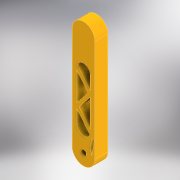
# Autodesk Inventor part: EslabonRodillaCadera
Saved by Autodesk Inventor 2021 (Build 250183000, 183)
## iProperties
Created: 2024-02-25
Part Number: EslabonRodillaCadera
Material: PLA
Document SubType Name: Modeling
Designer: Martin
Density: 1.27 g/cm^3
Appearance: PLA
Mass: 95.6941 g
Surface Area: 224.769 cm^2
Volume: 75.3497 cm^3
Author: Martin
Autodesk Inventor part; units mm, degrees
ref_plane "YZ Plane" through (0, 0, 0) normal (1, 0, 0) x (0, 1, 0)
ref_plane "XZ Plane" through (0, 0, 0) normal (0, 1, 0) x (-1, 0, 0)
ref_plane "XY Plane" through (0, 0, 0) normal (0, 0, 1) x (1, 0, 0)
sketch "Sketch1" plane through (0, 0, 0) normal (0, 0, 1) x (1, 0, 0)
  line L0 (0.0065, 157) -> (0.0065, 0) construction
  line L1 (-17.4935, 157) -> (-17.4935, 0)
  line L2 (17.5065, 0) -> (17.5065, 157)
  arc A0 (17.5065, 157) -> (-17.4935, 157) centre (0.0065, 157) ccw
  arc A1 (-17.4935, 0) -> (17.5065, 0) centre (0.0065, 0) ccw
  circle A2 centre (0.0065, 0) radius 11.1
  circle A3 centre (0.0065, 157) radius 7.5
  line L3 (4.0065, 157) -> (4.0065, 135)
  line L4 (4.0065, 135) -> (-3.9935, 135)
  line L5 (-3.9935, 135) -> (-3.9935, 157)
  line L6 (-3.9935, 157) -> (4.0065, 157)
  line L7 (0.0065, 157.5) -> (0.0065, -30.5)
  line L8 (0.0065, 157) -> (5.7519, 152.1791)
  line L9 (0.0065, 157) -> (0.0065, 149.5) construction
  arc A4 (5.7519, 152.1791) -> (4.0065, 147.4936) centre (13.9526, 146.4565) ccw
  line L10 (0.0065, 157) -> (-5.7388, 152.1791)
  arc A5 (-3.9935, 147.4936) -> (-5.7388, 152.1791) centre (-13.9395, 146.4565) ccw
  line L11 (0.0065, 157.5) -> (0.0065, 133.5) construction
  line L12 (4.0065, 157.5) -> (4.0065, 133.5)
  line L13 (-3.9935, 133.5) -> (-3.9935, 157.5)
  arc A6 (4.0065, 157.5) -> (-3.9935, 157.5) centre (0.0065, 157.5) ccw
  arc A7 (-3.9935, 133.5) -> (4.0065, 133.5) centre (0.0065, 133.5) ccw
  point P0 (0.0065, 157)
  point P1 (-3.9935, 147.4936)
  point P2 (0.0065, 145.5)
  dimension "d38" = 15
  dimension "d19" = 35
  dimension "d20" = 22.2
  dimension "d39" = 22
  dimension "d40" = 8
  dimension "d41" = 4
  dimension "d42" = 4
  dimension "d43" = 50
  dimension "d44" = 5
  dimension "d45" = 10
  dimension "d50" = 24
  dimension "d59" = 157
  constraints: 32 end point, 12 point on circle, 8 tangent, 7 centre point, 4 parallel, 2 point on line, 1 coincident, 1 equal length, 1 midpoint, 1 perpendicular, 1 vertical, 3 other
  measures "d19" diameter of A1
  measures "d20" diameter of A2
  measures "d39" distance of L5.start L5.end
  measures "d40" distance of L3.end L5.start
  measures "d41" distance between parallel lines of L5 L7
  measures "d42" distance between parallel lines of L7 L3
  measures "d43" angle of L9 L8
  measures "d44" distance of L8.end A4.end
  measures "d45" radius of A4
  measures "d50" distance of L7.start L11.end
  measures "d59" distance of L0.end L0.start
extrude "Extrusion1" add sketch "Sketch1" along normal mid plane 6
sketch "Sketch6" plane through (0, 0, 3) normal (0, 0, 1) x (1, 0, 0)
  arc A0 (-17.4935, 0) -> (17.5065, 0) centre (0.0065, 0) ccw projected
  line L0 (17.5065, 0) -> (17.5065, 157) projected
  arc A1 (17.5065, 157) -> (-17.4935, 157) centre (0.0065, 157) ccw projected
  line L1 (-17.4935, 157) -> (-17.4935, 0) projected
  arc A2 (-3.9935, 133.5) -> (4.0065, 133.5) centre (0.0065, 133.5) ccw projected
  line L2 (-3.9935, 133.5) -> (-3.9935, 147.4936) projected
  arc A3 (-3.9935, 147.4936) -> (-5.7388, 152.1791) centre (-13.9395, 146.4565) ccw projected
  arc A4 (5.7519, 152.1791) -> (-5.7388, 152.1791) centre (0.0065, 157) ccw projected
  arc A5 (5.7519, 152.1791) -> (4.0065, 147.4936) centre (13.9526, 146.4565) ccw projected
  line L3 (4.0065, 147.4936) -> (4.0065, 133.5) projected
  circle A6 centre (0.0065, 0) radius 11.1 projected
  point P0 (0, 0)
extrude "Extrusion4" add sketch "Sketch6" along normal blind 2 contours L1 A1 L0 A0 | L2 A3 A4 A5 L3 A2
sketch "Sketch7" plane through (0, 0, 5) normal (0, 0, 1) x (1, 0, 0)
  line L0 (0, 244.3) -> (0, -244.3) projected
  line L1 (17.5065, 0) -> (17.5065, 157) projected
  arc A0 (17.5065, 157) -> (-17.4935, 157) centre (0.0065, 157) ccw projected
  line L2 (-17.4935, 157) -> (-17.4935, 0) projected
  arc A1 (-17.4935, 0) -> (17.5065, 0) centre (0.0065, 0) ccw projected
  circle A2 centre (0.0065, 0) radius 11.1 projected
  circle A3 centre (0.0065, 0) radius 4.1
  point P0 (0, 0)
  point P1 (0, 11.1)
  point P2 (0, -11.1)
  point P3 (0, -17.5)
  point P4 (0, 174.5)
  dimension "d53" = 8.2
  constraints: 1 centre point, 1 coincident
  measures "d53" diameter of A3
extrude "Extrusion5" add sketch "Sketch7" along normal blind 12 contours A0 L1 A1 L0 A2 | L0 A2 A1 L2 A0 | A2 L0 A3 | L0 A3 A2
sketch "Sketch8" plane through (0, 0, 17) normal (0, 0, 1) x (1, 0, 0)
  line L0 (0, 108.776) -> (0, 32.1131) construction
  line L1 (12.4939, 108.776) -> (12.4939, 32.1131)
  line L2 (-12.4939, 32.1131) -> (-12.4939, 108.776)
  arc A0 (12.4939, 108.776) -> (-12.4939, 108.776) centre (0, 108.776) ccw
  arc A1 (-12.4939, 32.1131) -> (12.4939, 32.1131) centre (0, 32.1131) ccw
  line L3 (10.1612, 32.1131) -> (10.1612, 108.776)
  arc A2 (10.1612, 108.776) -> (-10.1612, 108.776) centre (0, 108.776) ccw
  line L4 (-10.1612, 108.776) -> (-10.1612, 32.1131)
  arc A3 (-10.1612, 32.1131) -> (10.1612, 32.1131) centre (0, 32.1131) ccw
  point P0 (0, 0)
  point P1 (0, 70.4445)
  constraints: 12 end point, 8 point on circle, 4 centre point, 4 tangent, 2 parallel, 1 midpoint, 1 vertical, 3 other
sketch "Sketch9" plane through (0, 0, -3) normal (0, 0, -1) x (-1, 0, 0)
  line L0 (-4.0065, 147.4936) -> (-4.0065, 133.5) projected
  arc A0 (-4.0065, 133.5) -> (3.9935, 133.5) centre (-0.0065, 133.5) ccw projected
  line L1 (3.9935, 133.5) -> (3.9935, 147.4936) projected
  arc A1 (5.7388, 152.1791) -> (3.9935, 147.4936) centre (13.9395, 146.4565) ccw projected
  arc A2 (5.7388, 152.1791) -> (-5.7519, 152.1791) centre (-0.0065, 157) ccw projected
  arc A3 (-4.0065, 147.4936) -> (-5.7519, 152.1791) centre (-13.9526, 146.4565) ccw projected
  line L2 (4.1935, 147.4832) -> (4.1935, 133.5)
  arc A4 (-4.2065, 133.5) -> (4.1935, 133.5) centre (-0.0065, 133.5) ccw
  line L3 (-4.2065, 133.5) -> (-4.2065, 147.4832)
  arc A5 (-4.2065, 147.4832) -> (-5.9109, 152.0574) centre (-13.9526, 146.4565) ccw
  arc A6 (5.8978, 152.0574) -> (-5.9109, 152.0574) centre (-0.0065, 157) ccw
  arc A7 (5.8978, 152.0574) -> (4.1935, 147.4832) centre (13.9395, 146.4565) ccw
  point P0 (0, 0)
  dimension "d60" = 0.2
  constraints: 8 point on circle, 4 centre point, 4 end point, 5 other
  measures "d60" radial gap between concentric circles of A1 A7
extrude "Extrusion7" cut sketch "Sketch9" against normal up to surface (6 mm away)
extrude "Extrusion9" cut sketch "Sketch8" against normal up to next contours A3 L4 A2 L3
sketch "Sketch11" plane through (0, 0, 17) normal (0, 0, 1) x (1, 0, 0)
  line L0 (10.9002, -1.9232) -> (15.7624, 25.6515)
  line L1 (10.9002, -1.9232) -> (38.9002, -1.9232) construction
  circle A0 centre (-0.0065, 0) radius 11.075
  circle A1 centre (-0.0065, 0) radius 12
  line L2 (16.7472, 25.4778) -> (12.092, -0.9232)
  line L3 (12.8079, 26.1724) -> (7.325, -4.9232)
  circle A2 centre (-0.0065, 0) radius 13
  circle A3 centre (-0.0065, 0) radius 10
  line L4 (12.8079, 26.1724) -> (16.7472, 25.4778)
  point P0 (0, 0)
  point P1 (0, 0)
  point P2 (9.7149, 8.631)
  point P3 (12.7213, 2.6461)
  dimension "d74" = 28
  dimension "d75" = 80
  dimension "d76" = 24
  dimension "d77" = 1
  dimension "d78" = 3
  dimension "d80" = 2
  constraints: 10 end point, 3 centre point, 1 coincident, 1 equal length, 1 horizontal, 4 other
  measures "d74" distance of L0.start L0.end
  measures "d75" angle of L1 L0
  measures "d76" diameter of A1
  measures "d77" distance between parallel lines of L0 L2
  measures "d78" distance between parallel lines of L0 L3
  measures "d80" radial gap between concentric circles of A1 A3
extrude "Extrusion10" cut sketch "Sketch11" against normal blind 8 contours A2 L3 L4 L0 | L0 L4 L2 A2
sketch "Sketch12" plane through (0, 0, 17) normal (0, 0, 1) x (1, 0, 0)
  arc A0 (12.7213, 2.6461) -> (9.7149, 8.631) centre (-0.0065, 0) ccw projected
  line L0 (9.7149, 8.631) -> (12.8079, 26.1724) projected
  line L1 (12.8079, 26.1724) -> (16.7472, 25.4778) projected
  line L2 (16.7472, 25.4778) -> (12.7213, 2.6461) projected
  line L3 (-10.1612, 32.1131) -> (-10.1612, 108.776) projected
  arc A1 (10.1612, 108.776) -> (-10.1612, 108.776) centre (0, 108.776) ccw projected
  line L4 (10.1612, 108.776) -> (10.1612, 32.1131) projected
  arc A2 (-10.1612, 32.1131) -> (10.1612, 32.1131) centre (0, 32.1131) ccw projected
  arc A3 (-17.4935, 0) -> (17.5065, 0) centre (0.0065, 0) ccw projected
  line L5 (17.5065, 0) -> (17.5065, 157) projected
  arc A4 (17.5065, 157) -> (-17.4935, 157) centre (0.0065, 157) ccw projected
  line L6 (-17.4935, 157) -> (-17.4935, 0) projected
  circle A5 centre (0.0065, 0) radius 4.1 projected
  line L7 (-10.1612, 108.776) -> (-10.1612, 32.1131) projected
  line L8 (-10.1612, 32.1131) -> (-10.1612, 57.6675)
  line L9 (10.1612, 108.776) -> (10.1612, 83.2216)
  line L10 (10.1612, 32.1131) -> (10.1612, 108.776) projected
  line L11 (10.1612, 32.1131) -> (-10.1612, 57.6675)
  line L12 (10.1612, 83.2216) -> (-10.1612, 57.6675)
  line L13 (10.1612, 83.2216) -> (-10.1612, 108.776)
  line L14 (12.1179, 84.7777) -> (-9.6047, 112.0926)
  line L15 (8.2046, 81.6655) -> (-12.1179, 107.2199)
  line L16 (8.2046, 84.7777) -> (-12.1179, 59.2236)
  line L17 (12.1179, 81.6655) -> (-8.2046, 56.1114)
  line L18 (12.1179, 33.6692) -> (-8.2046, 59.2235)
  line L19 (9.6047, 28.7964) -> (-12.1179, 56.1114)
  point P0 (0, 0)
  point P1 (10.1612, 87.2381)
  point P2 (-10.1612, 104.7595)
  point P3 (6.9671, 83.2216)
  point P4 (-10.1612, 61.6839)
  point P5 (-10.1612, 53.651)
  point P6 (10.1612, 36.1296)
  point P7 (-6.9671, 57.6675)
  point P8 (10.1612, 79.2051)
  dimension "d86" = 25.5543
  dimension "d87" = 25.5543
  dimension "d88" = 2.5
  dimension "d89" = 2.5
  dimension "d90" = 2.5
  dimension "d91" = 2.5
  dimension "d92" = 2.5
  dimension "d93" = 2.5
  constraints: 22 end point, 6 parallel, 2 point on circle, 2 point on line
  measures "d86" distance of L3.start L8.end
  measures "d87" distance of L4.start L9.end
  measures "d88" distance between parallel lines of L13 L14
  measures "d89" distance between parallel lines of L13 L15
  measures "d90" distance between parallel lines of L12 L16
  measures "d91" distance between parallel lines of L12 L17
  measures "d92" distance between parallel lines of L11 L18
  measures "d93" distance between parallel lines of L11 L19
extrude "Extrusion11" add sketch "Sketch12" against normal up to surface (20 mm away) contours L3 L11 A2 L19 | L12 L4 L17 L18 L11 | L3 L16 L15 L13 L12 | L13 A1 L14 L4
body "Solid1"
